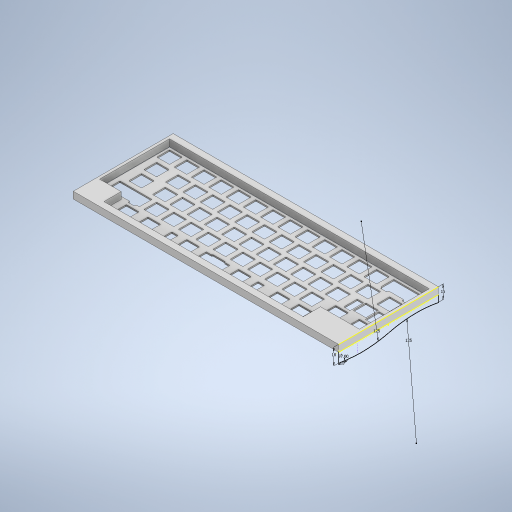
# Autodesk Inventor part: case
Saved by Autodesk Inventor 2023 (Build 270158000, 158)
## iProperties
Created: 2023-09-12
Part Number: case
Material: Generic
Document SubType Name: Modeling
Designer: Eric
Density: 1 g/cm^3
Appearance: Default
Author: Eric
Autodesk Inventor part; units mm, degrees
ref_plane "YZ Plane" through (0, 0, 0) normal (1, 0, 0) x (0, 1, 0)
ref_plane "XZ Plane" through (0, 0, 0) normal (0, 1, 0) x (-1, 0, 0)
ref_plane "XY Plane" through (0, 0, 0) normal (0, 0, 1) x (1, 0, 0)
sketch "Sketch1" plane through (0, 0, 0) normal (0, 1, 0) x (-1, 0, 0)
  line L0 (139.85, -45.1) -> (126.85, -45.1)
  line L1 (139.85, -31.1) -> (126.85, -31.1)
  line L2 (140.35, -44.6) -> (140.35, -31.6)
  line L3 (126.35, -44.6) -> (126.35, -31.6)
  arc A0 (139.85, -45.1) -> (140.35, -44.6) centre (139.85, -44.6) ccw
  arc A1 (126.35, -44.6) -> (126.85, -45.1) centre (126.85, -44.6) ccw
  arc A2 (140.35, -31.6) -> (139.85, -31.1) centre (139.85, -31.6) ccw
  arc A3 (126.85, -31.1) -> (126.35, -31.6) centre (126.85, -31.6) ccw
  line L4 (120.8, -45.1) -> (107.8, -45.1)
  line L5 (120.8, -31.1) -> (107.8, -31.1)
  line L6 (121.3, -44.6) -> (121.3, -31.6)
  line L7 (107.3, -44.6) -> (107.3, -31.6)
  arc A4 (120.8, -45.1) -> (121.3, -44.6) centre (120.8, -44.6) ccw
  arc A5 (107.3, -44.6) -> (107.8, -45.1) centre (107.8, -44.6) ccw
  arc A6 (121.3, -31.6) -> (120.8, -31.1) centre (120.8, -31.6) ccw
  arc A7 (107.8, -31.1) -> (107.3, -31.6) centre (107.8, -31.6) ccw
  line L8 (101.75, -45.1) -> (88.75, -45.1)
  line L9 (101.75, -31.1) -> (88.75, -31.1)
  line L10 (102.25, -44.6) -> (102.25, -31.6)
  line L11 (88.25, -44.6) -> (88.25, -31.6)
  arc A8 (101.75, -45.1) -> (102.25, -44.6) centre (101.75, -44.6) ccw
  arc A9 (88.25, -44.6) -> (88.75, -45.1) centre (88.75, -44.6) ccw
  arc A10 (102.25, -31.6) -> (101.75, -31.1) centre (101.75, -31.6) ccw
  arc A11 (88.75, -31.1) -> (88.25, -31.6) centre (88.75, -31.6) ccw
  line L12 (82.7, -45.1) -> (69.7, -45.1)
  line L13 (82.7, -31.1) -> (69.7, -31.1)
  line L14 (83.2, -44.6) -> (83.2, -31.6)
  line L15 (69.2, -44.6) -> (69.2, -31.6)
  arc A12 (82.7, -45.1) -> (83.2, -44.6) centre (82.7, -44.6) ccw
  arc A13 (69.2, -44.6) -> (69.7, -45.1) centre (69.7, -44.6) ccw
  arc A14 (83.2, -31.6) -> (82.7, -31.1) centre (82.7, -31.6) ccw
  arc A15 (69.7, -31.1) -> (69.2, -31.6) centre (69.7, -31.6) ccw
  line L16 (63.65, -45.1) -> (50.65, -45.1)
  line L17 (63.65, -31.1) -> (50.65, -31.1)
  line L18 (64.15, -44.6) -> (64.15, -31.6)
  line L19 (50.15, -44.6) -> (50.15, -31.6)
  arc A16 (63.65, -45.1) -> (64.15, -44.6) centre (63.65, -44.6) ccw
  arc A17 (50.15, -44.6) -> (50.65, -45.1) centre (50.65, -44.6) ccw
  arc A18 (64.15, -31.6) -> (63.65, -31.1) centre (63.65, -31.6) ccw
  arc A19 (50.65, -31.1) -> (50.15, -31.6) centre (50.65, -31.6) ccw
  line L20 (44.6, -45.1) -> (31.6, -45.1)
  line L21 (44.6, -31.1) -> (31.6, -31.1)
  line L22 (45.1, -44.6) -> (45.1, -31.6)
  line L23 (31.1, -44.6) -> (31.1, -31.6)
  arc A20 (44.6, -45.1) -> (45.1, -44.6) centre (44.6, -44.6) ccw
  arc A21 (31.1, -44.6) -> (31.6, -45.1) centre (31.6, -44.6) ccw
  arc A22 (45.1, -31.6) -> (44.6, -31.1) centre (44.6, -31.6) ccw
  arc A23 (31.6, -31.1) -> (31.1, -31.6) centre (31.6, -31.6) ccw
  line L24 (25.55, -45.1) -> (12.55, -45.1)
  line L25 (25.55, -31.1) -> (12.55, -31.1)
  line L26 (26.05, -44.6) -> (26.05, -31.6)
  line L27 (12.05, -44.6) -> (12.05, -31.6)
  arc A24 (25.55, -45.1) -> (26.05, -44.6) centre (25.55, -44.6) ccw
  arc A25 (12.05, -44.6) -> (12.55, -45.1) centre (12.55, -44.6) ccw
  arc A26 (26.05, -31.6) -> (25.55, -31.1) centre (25.55, -31.6) ccw
  arc A27 (12.55, -31.1) -> (12.05, -31.6) centre (12.55, -31.6) ccw
  line L28 (6.5, -45.1) -> (-6.5, -45.1)
  line L29 (6.5, -31.1) -> (-6.5, -31.1)
  line L30 (7, -44.6) -> (7, -31.6)
  line L31 (-7, -44.6) -> (-7, -31.6)
  arc A28 (6.5, -45.1) -> (7, -44.6) centre (6.5, -44.6) ccw
  arc A29 (-7, -44.6) -> (-6.5, -45.1) centre (-6.5, -44.6) ccw
  arc A30 (7, -31.6) -> (6.5, -31.1) centre (6.5, -31.6) ccw
  arc A31 (-6.5, -31.1) -> (-7, -31.6) centre (-6.5, -31.6) ccw
  line L32 (-12.55, -45.1) -> (-25.55, -45.1)
  line L33 (-12.55, -31.1) -> (-25.55, -31.1)
  line L34 (-12.05, -44.6) -> (-12.05, -31.6)
  line L35 (-26.05, -44.6) -> (-26.05, -31.6)
  arc A32 (-12.55, -45.1) -> (-12.05, -44.6) centre (-12.55, -44.6) ccw
  arc A33 (-26.05, -44.6) -> (-25.55, -45.1) centre (-25.55, -44.6) ccw
  arc A34 (-12.05, -31.6) -> (-12.55, -31.1) centre (-12.55, -31.6) ccw
  arc A35 (-25.55, -31.1) -> (-26.05, -31.6) centre (-25.55, -31.6) ccw
  line L36 (-31.6, -45.1) -> (-44.6, -45.1)
  line L37 (-31.6, -31.1) -> (-44.6, -31.1)
  line L38 (-31.1, -44.6) -> (-31.1, -31.6)
  line L39 (-45.1, -44.6) -> (-45.1, -31.6)
  arc A36 (-31.6, -45.1) -> (-31.1, -44.6) centre (-31.6, -44.6) ccw
  arc A37 (-45.1, -44.6) -> (-44.6, -45.1) centre (-44.6, -44.6) ccw
  arc A38 (-31.1, -31.6) -> (-31.6, -31.1) centre (-31.6, -31.6) ccw
  arc A39 (-44.6, -31.1) -> (-45.1, -31.6) centre (-44.6, -31.6) ccw
  line L40 (-50.65, -45.1) -> (-63.65, -45.1)
  line L41 (-50.65, -31.1) -> (-63.65, -31.1)
  line L42 (-50.15, -44.6) -> (-50.15, -31.6)
  line L43 (-64.15, -44.6) -> (-64.15, -31.6)
  arc A40 (-50.65, -45.1) -> (-50.15, -44.6) centre (-50.65, -44.6) ccw
  arc A41 (-64.15, -44.6) -> (-63.65, -45.1) centre (-63.65, -44.6) ccw
  arc A42 (-50.15, -31.6) -> (-50.65, -31.1) centre (-50.65, -31.6) ccw
  arc A43 (-63.65, -31.1) -> (-64.15, -31.6) centre (-63.65, -31.6) ccw
  line L44 (-69.7, -45.1) -> (-82.7, -45.1)
  line L45 (-69.7, -31.1) -> (-82.7, -31.1)
  line L46 (-69.2, -44.6) -> (-69.2, -31.6)
  line L47 (-83.2, -44.6) -> (-83.2, -31.6)
  arc A44 (-69.7, -45.1) -> (-69.2, -44.6) centre (-69.7, -44.6) ccw
  arc A45 (-83.2, -44.6) -> (-82.7, -45.1) centre (-82.7, -44.6) ccw
  arc A46 (-69.2, -31.6) -> (-69.7, -31.1) centre (-69.7, -31.6) ccw
  arc A47 (-82.7, -31.1) -> (-83.2, -31.6) centre (-82.7, -31.6) ccw
  line L48 (-88.75, -45.1) -> (-101.75, -45.1)
  line L49 (-88.75, -31.1) -> (-101.75, -31.1)
  line L50 (-88.25, -44.6) -> (-88.25, -31.6)
  line L51 (-102.25, -44.6) -> (-102.25, -31.6)
  arc A48 (-88.75, -45.1) -> (-88.25, -44.6) centre (-88.75, -44.6) ccw
  arc A49 (-102.25, -44.6) -> (-101.75, -45.1) centre (-101.75, -44.6) ccw
  arc A50 (-88.25, -31.6) -> (-88.75, -31.1) centre (-88.75, -31.6) ccw
  arc A51 (-101.75, -31.1) -> (-102.25, -31.6) centre (-101.75, -31.6) ccw
  line L52 (-117.325, -45.1) -> (-130.325, -45.1)
  line L53 (-117.325, -31.1) -> (-130.325, -31.1)
  line L54 (-108.887, -29.1) -> (-114.887, -29.1)
  line L55 (-108.387, -30.6) -> (-108.387, -29.6)
  line L56 (-115.387, -30.6) -> (-115.387, -29.6)
  arc A52 (-108.387, -29.6) -> (-108.887, -29.1) centre (-108.887, -29.6) ccw
  arc A53 (-114.887, -29.1) -> (-115.387, -29.6) centre (-114.887, -29.6) ccw
  line L57 (-132.763, -29.1) -> (-138.763, -29.1)
  line L58 (-132.263, -30.6) -> (-132.263, -29.6)
  line L59 (-139.263, -30.6) -> (-139.263, -29.6)
  arc A54 (-132.263, -29.6) -> (-132.763, -29.1) centre (-132.763, -29.6) ccw
  arc A55 (-138.763, -29.1) -> (-139.263, -29.6) centre (-138.763, -29.6) ccw
  line L60 (-107.8, -45.1) -> (-120.8, -45.1)
  line L61 (-107.3, -44.6) -> (-107.3, -31.6)
  arc A56 (-107.8, -45.1) -> (-107.3, -44.6) centre (-107.8, -44.6) ccw
  arc A57 (-107.3, -31.6) -> (-107.8, -31.1) centre (-107.8, -31.6) ccw
  line L62 (-126.85, -45.1) -> (-139.85, -45.1)
  line L63 (-140.35, -44.6) -> (-140.35, -31.6)
  arc A58 (-140.35, -44.6) -> (-139.85, -45.1) centre (-139.85, -44.6) ccw
  arc A59 (-139.85, -31.1) -> (-140.35, -31.6) centre (-139.85, -31.6) ccw
  line L64 (135.0875, -26.05) -> (122.0875, -26.05)
  line L65 (135.0875, -12.05) -> (122.0875, -12.05)
  line L66 (135.5875, -25.55) -> (135.5875, -12.55)
  line L67 (121.5875, -25.55) -> (121.5875, -12.55)
  arc A60 (135.0875, -26.05) -> (135.5875, -25.55) centre (135.0875, -25.55) ccw
  arc A61 (121.5875, -25.55) -> (122.0875, -26.05) centre (122.0875, -25.55) ccw
  arc A62 (135.5875, -12.55) -> (135.0875, -12.05) centre (135.0875, -12.55) ccw
  arc A63 (122.0875, -12.05) -> (121.5875, -12.55) centre (122.0875, -12.55) ccw
  line L68 (111.275, -26.05) -> (98.275, -26.05)
  line L69 (111.275, -12.05) -> (98.275, -12.05)
  line L70 (111.775, -25.55) -> (111.775, -12.55)
  line L71 (97.775, -25.55) -> (97.775, -12.55)
  arc A64 (111.275, -26.05) -> (111.775, -25.55) centre (111.275, -25.55) ccw
  arc A65 (97.775, -25.55) -> (98.275, -26.05) centre (98.275, -25.55) ccw
  arc A66 (111.775, -12.55) -> (111.275, -12.05) centre (111.275, -12.55) ccw
  arc A67 (98.275, -12.05) -> (97.775, -12.55) centre (98.275, -12.55) ccw
  line L72 (92.225, -26.05) -> (79.225, -26.05)
  line L73 (92.225, -12.05) -> (79.225, -12.05)
  line L74 (92.725, -25.55) -> (92.725, -12.55)
  line L75 (78.725, -25.55) -> (78.725, -12.55)
  arc A68 (92.225, -26.05) -> (92.725, -25.55) centre (92.225, -25.55) ccw
  arc A69 (78.725, -25.55) -> (79.225, -26.05) centre (79.225, -25.55) ccw
  arc A70 (92.725, -12.55) -> (92.225, -12.05) centre (92.225, -12.55) ccw
  arc A71 (79.225, -12.05) -> (78.725, -12.55) centre (79.225, -12.55) ccw
  line L76 (73.175, -26.05) -> (60.175, -26.05)
  line L77 (73.175, -12.05) -> (60.175, -12.05)
  line L78 (73.675, -25.55) -> (73.675, -12.55)
  line L79 (59.675, -25.55) -> (59.675, -12.55)
  arc A72 (73.175, -26.05) -> (73.675, -25.55) centre (73.175, -25.55) ccw
  arc A73 (59.675, -25.55) -> (60.175, -26.05) centre (60.175, -25.55) ccw
  arc A74 (73.675, -12.55) -> (73.175, -12.05) centre (73.175, -12.55) ccw
  arc A75 (60.175, -12.05) -> (59.675, -12.55) centre (60.175, -12.55) ccw
  line L80 (54.125, -26.05) -> (41.125, -26.05)
  line L81 (54.125, -12.05) -> (41.125, -12.05)
  line L82 (54.625, -25.55) -> (54.625, -12.55)
  line L83 (40.625, -25.55) -> (40.625, -12.55)
  arc A76 (54.125, -26.05) -> (54.625, -25.55) centre (54.125, -25.55) ccw
  arc A77 (40.625, -25.55) -> (41.125, -26.05) centre (41.125, -25.55) ccw
  arc A78 (54.625, -12.55) -> (54.125, -12.05) centre (54.125, -12.55) ccw
  arc A79 (41.125, -12.05) -> (40.625, -12.55) centre (41.125, -12.55) ccw
  line L84 (35.075, -26.05) -> (22.075, -26.05)
  line L85 (35.075, -12.05) -> (22.075, -12.05)
  line L86 (35.575, -25.55) -> (35.575, -12.55)
  line L87 (21.575, -25.55) -> (21.575, -12.55)
  arc A80 (35.075, -26.05) -> (35.575, -25.55) centre (35.075, -25.55) ccw
  arc A81 (21.575, -25.55) -> (22.075, -26.05) centre (22.075, -25.55) ccw
  arc A82 (35.575, -12.55) -> (35.075, -12.05) centre (35.075, -12.55) ccw
  arc A83 (22.075, -12.05) -> (21.575, -12.55) centre (22.075, -12.55) ccw
  line L88 (16.025, -26.05) -> (3.025, -26.05)
  line L89 (16.025, -12.05) -> (3.025, -12.05)
  line L90 (16.525, -25.55) -> (16.525, -12.55)
  line L91 (2.525, -25.55) -> (2.525, -12.55)
  arc A84 (16.025, -26.05) -> (16.525, -25.55) centre (16.025, -25.55) ccw
  arc A85 (2.525, -25.55) -> (3.025, -26.05) centre (3.025, -25.55) ccw
  arc A86 (16.525, -12.55) -> (16.025, -12.05) centre (16.025, -12.55) ccw
  arc A87 (3.025, -12.05) -> (2.525, -12.55) centre (3.025, -12.55) ccw
  line L92 (-3.025, -26.05) -> (-16.025, -26.05)
  line L93 (-3.025, -12.05) -> (-16.025, -12.05)
  line L94 (-2.525, -25.55) -> (-2.525, -12.55)
  line L95 (-16.525, -25.55) -> (-16.525, -12.55)
  arc A88 (-3.025, -26.05) -> (-2.525, -25.55) centre (-3.025, -25.55) ccw
  arc A89 (-16.525, -25.55) -> (-16.025, -26.05) centre (-16.025, -25.55) ccw
  arc A90 (-2.525, -12.55) -> (-3.025, -12.05) centre (-3.025, -12.55) ccw
  arc A91 (-16.025, -12.05) -> (-16.525, -12.55) centre (-16.025, -12.55) ccw
  line L96 (-22.075, -26.05) -> (-35.075, -26.05)
  line L97 (-22.075, -12.05) -> (-35.075, -12.05)
  line L98 (-21.575, -25.55) -> (-21.575, -12.55)
  line L99 (-35.575, -25.55) -> (-35.575, -12.55)
  arc A92 (-22.075, -26.05) -> (-21.575, -25.55) centre (-22.075, -25.55) ccw
  arc A93 (-35.575, -25.55) -> (-35.075, -26.05) centre (-35.075, -25.55) ccw
  arc A94 (-21.575, -12.55) -> (-22.075, -12.05) centre (-22.075, -12.55) ccw
  arc A95 (-35.075, -12.05) -> (-35.575, -12.55) centre (-35.075, -12.55) ccw
  line L100 (-41.125, -26.05) -> (-54.125, -26.05)
  line L101 (-41.125, -12.05) -> (-54.125, -12.05)
  line L102 (-40.625, -25.55) -> (-40.625, -12.55)
  line L103 (-54.625, -25.55) -> (-54.625, -12.55)
  arc A96 (-41.125, -26.05) -> (-40.625, -25.55) centre (-41.125, -25.55) ccw
  arc A97 (-54.625, -25.55) -> (-54.125, -26.05) centre (-54.125, -25.55) ccw
  arc A98 (-40.625, -12.55) -> (-41.125, -12.05) centre (-41.125, -12.55) ccw
  arc A99 (-54.125, -12.05) -> (-54.625, -12.55) centre (-54.125, -12.55) ccw
  line L104 (-60.175, -26.05) -> (-73.175, -26.05)
  line L105 (-60.175, -12.05) -> (-73.175, -12.05)
  line L106 (-59.675, -25.55) -> (-59.675, -12.55)
  line L107 (-73.675, -25.55) -> (-73.675, -12.55)
  arc A100 (-60.175, -26.05) -> (-59.675, -25.55) centre (-60.175, -25.55) ccw
  arc A101 (-73.675, -25.55) -> (-73.175, -26.05) centre (-73.175, -25.55) ccw
  arc A102 (-59.675, -12.55) -> (-60.175, -12.05) centre (-60.175, -12.55) ccw
  arc A103 (-73.175, -12.05) -> (-73.675, -12.55) centre (-73.175, -12.55) ccw
  line L108 (-79.225, -26.05) -> (-92.225, -26.05)
  line L109 (-79.225, -12.05) -> (-92.225, -12.05)
  line L110 (-78.725, -25.55) -> (-78.725, -12.55)
  line L111 (-92.725, -25.55) -> (-92.725, -12.55)
  arc A104 (-79.225, -26.05) -> (-78.725, -25.55) centre (-79.225, -25.55) ccw
  arc A105 (-92.725, -25.55) -> (-92.225, -26.05) centre (-92.225, -25.55) ccw
  arc A106 (-78.725, -12.55) -> (-79.225, -12.05) centre (-79.225, -12.55) ccw
  arc A107 (-92.225, -12.05) -> (-92.725, -12.55) centre (-92.225, -12.55) ccw
  line L112 (-98.275, -26.05) -> (-111.275, -26.05)
  line L113 (-98.275, -12.05) -> (-111.275, -12.05)
  line L114 (-97.775, -25.55) -> (-97.775, -12.55)
  line L115 (-111.775, -25.55) -> (-111.775, -12.55)
  arc A108 (-98.275, -26.05) -> (-97.775, -25.55) centre (-98.275, -25.55) ccw
  arc A109 (-111.775, -25.55) -> (-111.275, -26.05) centre (-111.275, -25.55) ccw
  arc A110 (-97.775, -12.55) -> (-98.275, -12.05) centre (-98.275, -12.55) ccw
  arc A111 (-111.275, -12.05) -> (-111.775, -12.55) centre (-111.275, -12.55) ccw
  line L116 (-122.0875, -26.05) -> (-135.0875, -26.05)
  line L117 (-122.0875, -12.05) -> (-135.0875, -12.05)
  line L118 (-121.5875, -25.55) -> (-121.5875, -12.55)
  line L119 (-135.5875, -25.55) -> (-135.5875, -12.55)
  arc A112 (-122.0875, -26.05) -> (-121.5875, -25.55) centre (-122.0875, -25.55) ccw
  arc A113 (-135.5875, -25.55) -> (-135.0875, -26.05) centre (-135.0875, -25.55) ccw
  arc A114 (-121.5875, -12.55) -> (-122.0875, -12.05) centre (-122.0875, -12.55) ccw
  arc A115 (-135.0875, -12.05) -> (-135.5875, -12.55) centre (-135.0875, -12.55) ccw
  line L120 (132.7062, -7) -> (119.7062, -7)
  line L121 (132.7062, 7) -> (119.7062, 7)
  line L122 (133.2062, -6.5) -> (133.2062, 6.5)
  line L123 (119.2062, -6.5) -> (119.2062, 6.5)
  arc A116 (132.7062, -7) -> (133.2062, -6.5) centre (132.7062, -6.5) ccw
  arc A117 (119.2062, -6.5) -> (119.7062, -7) centre (119.7062, -6.5) ccw
  arc A118 (133.2062, 6.5) -> (132.7062, 7) centre (132.7062, 6.5) ccw
  arc A119 (119.7062, 7) -> (119.2062, 6.5) centre (119.7062, 6.5) ccw
  line L124 (106.5125, -7) -> (93.5125, -7)
  line L125 (106.5125, 7) -> (93.5125, 7)
  line L126 (107.0125, -6.5) -> (107.0125, 6.5)
  line L127 (93.0125, -6.5) -> (93.0125, 6.5)
  arc A120 (106.5125, -7) -> (107.0125, -6.5) centre (106.5125, -6.5) ccw
  arc A121 (93.0125, -6.5) -> (93.5125, -7) centre (93.5125, -6.5) ccw
  arc A122 (107.0125, 6.5) -> (106.5125, 7) centre (106.5125, 6.5) ccw
  arc A123 (93.5125, 7) -> (93.0125, 6.5) centre (93.5125, 6.5) ccw
  line L128 (87.4625, -7) -> (74.4625, -7)
  line L129 (87.4625, 7) -> (74.4625, 7)
  line L130 (87.9625, -6.5) -> (87.9625, 6.5)
  line L131 (73.9625, -6.5) -> (73.9625, 6.5)
  arc A124 (87.4625, -7) -> (87.9625, -6.5) centre (87.4625, -6.5) ccw
  arc A125 (73.9625, -6.5) -> (74.4625, -7) centre (74.4625, -6.5) ccw
  arc A126 (87.9625, 6.5) -> (87.4625, 7) centre (87.4625, 6.5) ccw
  arc A127 (74.4625, 7) -> (73.9625, 6.5) centre (74.4625, 6.5) ccw
  line L132 (68.4125, -7) -> (55.4125, -7)
  line L133 (68.4125, 7) -> (55.4125, 7)
  line L134 (68.9125, -6.5) -> (68.9125, 6.5)
  line L135 (54.9125, -6.5) -> (54.9125, 6.5)
  arc A128 (68.4125, -7) -> (68.9125, -6.5) centre (68.4125, -6.5) ccw
  arc A129 (54.9125, -6.5) -> (55.4125, -7) centre (55.4125, -6.5) ccw
  arc A130 (68.9125, 6.5) -> (68.4125, 7) centre (68.4125, 6.5) ccw
  arc A131 (55.4125, 7) -> (54.9125, 6.5) centre (55.4125, 6.5) ccw
  line L136 (49.3625, -7) -> (36.3625, -7)
  line L137 (49.3625, 7) -> (36.3625, 7)
  line L138 (49.8625, -6.5) -> (49.8625, 6.5)
  line L139 (35.8625, -6.5) -> (35.8625, 6.5)
  arc A132 (49.3625, -7) -> (49.8625, -6.5) centre (49.3625, -6.5) ccw
  arc A133 (35.8625, -6.5) -> (36.3625, -7) centre (36.3625, -6.5) ccw
  arc A134 (49.8625, 6.5) -> (49.3625, 7) centre (49.3625, 6.5) ccw
  arc A135 (36.3625, 7) -> (35.8625, 6.5) centre (36.3625, 6.5) ccw
  line L140 (30.3125, -7) -> (17.3125, -7)
  line L141 (30.3125, 7) -> (17.3125, 7)
  line L142 (30.8125, -6.5) -> (30.8125, 6.5)
  line L143 (16.8125, -6.5) -> (16.8125, 6.5)
  arc A136 (30.3125, -7) -> (30.8125, -6.5) centre (30.3125, -6.5) ccw
  arc A137 (16.8125, -6.5) -> (17.3125, -7) centre (17.3125, -6.5) ccw
  arc A138 (30.8125, 6.5) -> (30.3125, 7) centre (30.3125, 6.5) ccw
  arc A139 (17.3125, 7) -> (16.8125, 6.5) centre (17.3125, 6.5) ccw
  line L144 (11.2625, -7) -> (-1.7375, -7)
  line L145 (11.2625, 7) -> (-1.7375, 7)
  line L146 (11.7625, -6.5) -> (11.7625, 6.5)
  line L147 (-2.2375, -6.5) -> (-2.2375, 6.5)
  arc A140 (11.2625, -7) -> (11.7625, -6.5) centre (11.2625, -6.5) ccw
  arc A141 (-2.2375, -6.5) -> (-1.7375, -7) centre (-1.7375, -6.5) ccw
  arc A142 (11.7625, 6.5) -> (11.2625, 7) centre (11.2625, 6.5) ccw
  arc A143 (-1.7375, 7) -> (-2.2375, 6.5) centre (-1.7375, 6.5) ccw
  line L148 (-7.7875, -7) -> (-20.7875, -7)
  line L149 (-7.7875, 7) -> (-20.7875, 7)
  line L150 (-7.2875, -6.5) -> (-7.2875, 6.5)
  line L151 (-21.2875, -6.5) -> (-21.2875, 6.5)
  arc A144 (-7.7875, -7) -> (-7.2875, -6.5) centre (-7.7875, -6.5) ccw
  arc A145 (-21.2875, -6.5) -> (-20.7875, -7) centre (-20.7875, -6.5) ccw
  arc A146 (-7.2875, 6.5) -> (-7.7875, 7) centre (-7.7875, 6.5) ccw
  arc A147 (-20.7875, 7) -> (-21.2875, 6.5) centre (-20.7875, 6.5) ccw
  line L152 (-26.8375, -7) -> (-39.8375, -7)
  line L153 (-26.8375, 7) -> (-39.8375, 7)
  line L154 (-26.3375, -6.5) -> (-26.3375, 6.5)
  line L155 (-40.3375, -6.5) -> (-40.3375, 6.5)
  arc A148 (-26.8375, -7) -> (-26.3375, -6.5) centre (-26.8375, -6.5) ccw
  arc A149 (-40.3375, -6.5) -> (-39.8375, -7) centre (-39.8375, -6.5) ccw
  arc A150 (-26.3375, 6.5) -> (-26.8375, 7) centre (-26.8375, 6.5) ccw
  arc A151 (-39.8375, 7) -> (-40.3375, 6.5) centre (-39.8375, 6.5) ccw
  line L156 (-45.8875, -7) -> (-58.8875, -7)
  line L157 (-45.8875, 7) -> (-58.8875, 7)
  line L158 (-45.3875, -6.5) -> (-45.3875, 6.5)
  line L159 (-59.3875, -6.5) -> (-59.3875, 6.5)
  arc A152 (-45.8875, -7) -> (-45.3875, -6.5) centre (-45.8875, -6.5) ccw
  arc A153 (-59.3875, -6.5) -> (-58.8875, -7) centre (-58.8875, -6.5) ccw
  arc A154 (-45.3875, 6.5) -> (-45.8875, 7) centre (-45.8875, 6.5) ccw
  arc A155 (-58.8875, 7) -> (-59.3875, 6.5) centre (-58.8875, 6.5) ccw
  line L160 (-64.9375, -7) -> (-77.9375, -7)
  line L161 (-64.9375, 7) -> (-77.9375, 7)
  line L162 (-64.4375, -6.5) -> (-64.4375, 6.5)
  line L163 (-78.4375, -6.5) -> (-78.4375, 6.5)
  arc A156 (-64.9375, -7) -> (-64.4375, -6.5) centre (-64.9375, -6.5) ccw
  arc A157 (-78.4375, -6.5) -> (-77.9375, -7) centre (-77.9375, -6.5) ccw
  arc A158 (-64.4375, 6.5) -> (-64.9375, 7) centre (-64.9375, 6.5) ccw
  arc A159 (-77.9375, 7) -> (-78.4375, 6.5) centre (-77.9375, 6.5) ccw
  line L164 (-83.9875, -7) -> (-96.9875, -7)
  line L165 (-83.9875, 7) -> (-96.9875, 7)
  line L166 (-83.4875, -6.5) -> (-83.4875, 6.5)
  line L167 (-97.4875, -6.5) -> (-97.4875, 6.5)
  arc A160 (-83.9875, -7) -> (-83.4875, -6.5) centre (-83.9875, -6.5) ccw
  arc A161 (-97.4875, -6.5) -> (-96.9875, -7) centre (-96.9875, -6.5) ccw
  arc A162 (-83.4875, 6.5) -> (-83.9875, 7) centre (-83.9875, 6.5) ccw
  arc A163 (-96.9875, 7) -> (-97.4875, 6.5) centre (-96.9875, 6.5) ccw
  line L168 (-114.9438, -7) -> (-127.9438, -7)
  line L169 (-114.9437, 7) -> (-127.9437, 7)
  line L170 (-114.4438, -6.5) -> (-114.4437, 6.5)
  line L171 (-128.4438, -6.5) -> (-128.4438, 6.5)
  arc A164 (-114.9438, -7) -> (-114.4438, -6.5) centre (-114.9438, -6.5) ccw
  arc A165 (-128.4438, -6.5) -> (-127.9438, -7) centre (-127.9438, -6.5) ccw
  arc A166 (-114.4437, 6.5) -> (-114.9437, 7) centre (-114.9437, 6.5) ccw
  arc A167 (-127.9437, 7) -> (-128.4438, 6.5) centre (-127.9438, 6.5) ccw
  line L172 (-106.5058, -6) -> (-112.5058, -6)
  line L173 (-106.5058, 9) -> (-112.5057, 9)
  line L174 (-106.0058, -5.5) -> (-106.0058, 8.5)
  line L175 (-113.0058, -5.5) -> (-113.0057, 8.5)
  arc A168 (-106.5058, -6) -> (-106.0058, -5.5) centre (-106.5058, -5.5) ccw
  arc A169 (-113.0058, -5.5) -> (-112.5058, -6) centre (-112.5058, -5.5) ccw
  arc A170 (-106.0058, 8.5) -> (-106.5058, 9) centre (-106.5058, 8.5) ccw
  arc A171 (-112.5057, 9) -> (-113.0057, 8.5) centre (-112.5057, 8.5) ccw
  line L176 (-130.3817, -6) -> (-136.3817, -6)
  line L177 (-130.3818, 9) -> (-136.3818, 9)
  line L178 (-129.8818, -5.5) -> (-129.8818, 8.5)
  line L179 (-136.8817, -5.5) -> (-136.8818, 8.5)
  arc A172 (-130.3817, -6) -> (-129.8818, -5.5) centre (-130.3818, -5.5) ccw
  arc A173 (-136.8817, -5.5) -> (-136.3817, -6) centre (-136.3817, -5.5) ccw
  arc A174 (-129.8818, 8.5) -> (-130.3818, 9) centre (-130.3818, 8.5) ccw
  arc A175 (-136.3818, 9) -> (-136.8818, 8.5) centre (-136.3818, 8.5) ccw
  line L180 (127.9437, 12.05) -> (114.9437, 12.05)
  line L181 (127.9437, 26.05) -> (114.9437, 26.05)
  line L182 (136.3817, 28.05) -> (130.3817, 28.05)
  line L183 (136.8817, 26.55) -> (136.8817, 27.55)
  line L184 (129.8817, 26.55) -> (129.8817, 27.55)
  arc A176 (136.8817, 27.55) -> (136.3817, 28.05) centre (136.3817, 27.55) ccw
  arc A177 (130.3817, 28.05) -> (129.8817, 27.55) centre (130.3817, 27.55) ccw
  line L185 (112.5057, 28.05) -> (106.5058, 28.05)
  line L186 (113.0057, 26.55) -> (113.0057, 27.55)
  line L187 (106.0057, 26.55) -> (106.0057, 27.55)
  arc A178 (113.0057, 27.55) -> (112.5057, 28.05) centre (112.5057, 27.55) ccw
  arc A179 (106.5058, 28.05) -> (106.0057, 27.55) centre (106.5058, 27.55) ccw
  line L188 (137.4688, 12.05) -> (124.4687, 12.05)
  line L189 (137.9687, 12.55) -> (137.9687, 25.55)
  arc A180 (137.4688, 12.05) -> (137.9687, 12.55) centre (137.4687, 12.55) ccw
  arc A181 (137.9687, 25.55) -> (137.4688, 26.05) centre (137.4688, 25.55) ccw
  line L190 (116.0375, 12.05) -> (103.0375, 12.05)
  line L191 (102.5375, 12.55) -> (102.5375, 25.55)
  arc A182 (102.5375, 12.55) -> (103.0375, 12.05) centre (103.0375, 12.55) ccw
  arc A183 (103.0375, 26.05) -> (102.5375, 25.55) centre (103.0375, 25.55) ccw
  line L192 (96.9875, 12.05) -> (83.9875, 12.05)
  line L193 (96.9875, 26.05) -> (83.9875, 26.05)
  line L194 (97.4875, 12.55) -> (97.4875, 25.55)
  line L195 (83.4875, 12.55) -> (83.4875, 25.55)
  arc A184 (96.9875, 12.05) -> (97.4875, 12.55) centre (96.9875, 12.55) ccw
  arc A185 (83.4875, 12.55) -> (83.9875, 12.05) centre (83.9875, 12.55) ccw
  arc A186 (97.4875, 25.55) -> (96.9875, 26.05) centre (96.9875, 25.55) ccw
  arc A187 (83.9875, 26.05) -> (83.4875, 25.55) centre (83.9875, 25.55) ccw
  line L196 (77.9375, 12.05) -> (64.9375, 12.05)
  line L197 (77.9375, 26.05) -> (64.9375, 26.05)
  line L198 (78.4375, 12.55) -> (78.4375, 25.55)
  line L199 (64.4375, 12.55) -> (64.4375, 25.55)
  arc A188 (77.9375, 12.05) -> (78.4375, 12.55) centre (77.9375, 12.55) ccw
  arc A189 (64.4375, 12.55) -> (64.9375, 12.05) centre (64.9375, 12.55) ccw
  arc A190 (78.4375, 25.55) -> (77.9375, 26.05) centre (77.9375, 25.55) ccw
  arc A191 (64.9375, 26.05) -> (64.4375, 25.55) centre (64.9375, 25.55) ccw
  line L200 (58.8875, 12.05) -> (45.8875, 12.05)
  line L201 (58.8875, 26.05) -> (45.8875, 26.05)
  line L202 (59.3875, 12.55) -> (59.3875, 25.55)
  line L203 (45.3875, 12.55) -> (45.3875, 25.55)
  arc A192 (58.8875, 12.05) -> (59.3875, 12.55) centre (58.8875, 12.55) ccw
  arc A193 (45.3875, 12.55) -> (45.8875, 12.05) centre (45.8875, 12.55) ccw
  arc A194 (59.3875, 25.55) -> (58.8875, 26.05) centre (58.8875, 25.55) ccw
  arc A195 (45.8875, 26.05) -> (45.3875, 25.55) centre (45.8875, 25.55) ccw
  line L204 (39.8375, 12.05) -> (26.8375, 12.05)
  line L205 (39.8375, 26.05) -> (26.8375, 26.05)
  line L206 (40.3375, 12.55) -> (40.3375, 25.55)
  line L207 (26.3375, 12.55) -> (26.3375, 25.55)
  arc A196 (39.8375, 12.05) -> (40.3375, 12.55) centre (39.8375, 12.55) ccw
  arc A197 (26.3375, 12.55) -> (26.8375, 12.05) centre (26.8375, 12.55) ccw
  arc A198 (40.3375, 25.55) -> (39.8375, 26.05) centre (39.8375, 25.55) ccw
  arc A199 (26.8375, 26.05) -> (26.3375, 25.55) centre (26.8375, 25.55) ccw
  line L208 (20.7875, 12.05) -> (7.7875, 12.05)
  line L209 (20.7875, 26.05) -> (7.7875, 26.05)
  line L210 (21.2875, 12.55) -> (21.2875, 25.55)
  line L211 (7.2875, 12.55) -> (7.2875, 25.55)
  arc A200 (20.7875, 12.05) -> (21.2875, 12.55) centre (20.7875, 12.55) ccw
  arc A201 (7.2875, 12.55) -> (7.7875, 12.05) centre (7.7875, 12.55) ccw
  arc A202 (21.2875, 25.55) -> (20.7875, 26.05) centre (20.7875, 25.55) ccw
  arc A203 (7.7875, 26.05) -> (7.2875, 25.55) centre (7.7875, 25.55) ccw
  line L212 (1.7375, 12.05) -> (-11.2625, 12.05)
  line L213 (1.7375, 26.05) -> (-11.2625, 26.05)
  line L214 (2.2375, 12.55) -> (2.2375, 25.55)
  line L215 (-11.7625, 12.55) -> (-11.7625, 25.55)
  arc A204 (1.7375, 12.05) -> (2.2375, 12.55) centre (1.7375, 12.55) ccw
  arc A205 (-11.7625, 12.55) -> (-11.2625, 12.05) centre (-11.2625, 12.55) ccw
  arc A206 (2.2375, 25.55) -> (1.7375, 26.05) centre (1.7375, 25.55) ccw
  arc A207 (-11.2625, 26.05) -> (-11.7625, 25.55) centre (-11.2625, 25.55) ccw
  line L216 (-17.3125, 12.05) -> (-30.3125, 12.05)
  line L217 (-17.3125, 26.05) -> (-30.3125, 26.05)
  line L218 (-16.8125, 12.55) -> (-16.8125, 25.55)
  line L219 (-30.8125, 12.55) -> (-30.8125, 25.55)
  arc A208 (-17.3125, 12.05) -> (-16.8125, 12.55) centre (-17.3125, 12.55) ccw
  arc A209 (-30.8125, 12.55) -> (-30.3125, 12.05) centre (-30.3125, 12.55) ccw
  arc A210 (-16.8125, 25.55) -> (-17.3125, 26.05) centre (-17.3125, 25.55) ccw
  arc A211 (-30.3125, 26.05) -> (-30.8125, 25.55) centre (-30.3125, 25.55) ccw
  line L220 (-36.3625, 12.05) -> (-49.3625, 12.05)
  line L221 (-36.3625, 26.05) -> (-49.3625, 26.05)
  line L222 (-35.8625, 12.55) -> (-35.8625, 25.55)
  line L223 (-49.8625, 12.55) -> (-49.8625, 25.55)
  arc A212 (-36.3625, 12.05) -> (-35.8625, 12.55) centre (-36.3625, 12.55) ccw
  arc A213 (-49.8625, 12.55) -> (-49.3625, 12.05) centre (-49.3625, 12.55) ccw
  arc A214 (-35.8625, 25.55) -> (-36.3625, 26.05) centre (-36.3625, 25.55) ccw
  arc A215 (-49.3625, 26.05) -> (-49.8625, 25.55) centre (-49.3625, 25.55) ccw
  line L224 (-55.4125, 12.05) -> (-68.4125, 12.05)
  line L225 (-55.4125, 26.05) -> (-68.4125, 26.05)
  line L226 (-54.9125, 12.55) -> (-54.9125, 25.55)
  line L227 (-68.9125, 12.55) -> (-68.9125, 25.55)
  arc A216 (-55.4125, 12.05) -> (-54.9125, 12.55) centre (-55.4125, 12.55) ccw
  arc A217 (-68.9125, 12.55) -> (-68.4125, 12.05) centre (-68.4125, 12.55) ccw
  arc A218 (-54.9125, 25.55) -> (-55.4125, 26.05) centre (-55.4125, 25.55) ccw
  arc A219 (-68.4125, 26.05) -> (-68.9125, 25.55) centre (-68.4125, 25.55) ccw
  line L228 (-74.4625, 12.05) -> (-87.4625, 12.05)
  line L229 (-74.4625, 26.05) -> (-87.4625, 26.05)
  line L230 (-73.9625, 12.55) -> (-73.9625, 25.55)
  line L231 (-87.9625, 12.55) -> (-87.9625, 25.55)
  arc A220 (-74.4625, 12.05) -> (-73.9625, 12.55) centre (-74.4625, 12.55) ccw
  arc A221 (-87.9625, 12.55) -> (-87.4625, 12.05) centre (-87.4625, 12.55) ccw
  arc A222 (-73.9625, 25.55) -> (-74.4625, 26.05) centre (-74.4625, 25.55) ccw
  arc A223 (-87.4625, 26.05) -> (-87.9625, 25.55) centre (-87.4625, 25.55) ccw
  line L232 (-100.6562, 12.05) -> (-113.6563, 12.05)
  line L233 (-100.6562, 26.05) -> (-113.6562, 26.05)
  line L234 (-100.1563, 12.55) -> (-100.1562, 25.55)
  line L235 (-114.1563, 12.55) -> (-114.1562, 25.55)
  arc A224 (-100.6562, 12.05) -> (-100.1563, 12.55) centre (-100.6563, 12.55) ccw
  arc A225 (-114.1563, 12.55) -> (-113.6563, 12.05) centre (-113.6563, 12.55) ccw
  arc A226 (-100.1562, 25.55) -> (-100.6562, 26.05) centre (-100.6562, 25.55) ccw
  arc A227 (-113.6562, 26.05) -> (-114.1562, 25.55) centre (-113.6562, 25.55) ccw
  line L236 (-126.85, 12.05) -> (-139.85, 12.05)
  line L237 (-126.85, 26.05) -> (-139.85, 26.05)
  line L238 (-126.35, 12.55) -> (-126.35, 25.55)
  line L239 (-140.35, 12.55) -> (-140.35, 25.55)
  arc A228 (-126.85, 12.05) -> (-126.35, 12.55) centre (-126.85, 12.55) ccw
  arc A229 (-140.35, 12.55) -> (-139.85, 12.05) centre (-139.85, 12.55) ccw
  arc A230 (-126.35, 25.55) -> (-126.85, 26.05) centre (-126.85, 25.55) ccw
  arc A231 (-139.85, 26.05) -> (-140.35, 25.55) centre (-139.85, 25.55) ccw
  line L240 (111.275, 31.1) -> (98.275, 31.1)
  line L241 (111.275, 45.1) -> (98.275, 45.1)
  line L242 (111.775, 31.6) -> (111.775, 44.6)
  line L243 (97.775, 31.6) -> (97.775, 44.6)
  arc A232 (111.275, 31.1) -> (111.775, 31.6) centre (111.275, 31.6) ccw
  arc A233 (97.775, 31.6) -> (98.275, 31.1) centre (98.275, 31.6) ccw
  arc A234 (111.775, 44.6) -> (111.275, 45.1) centre (111.275, 44.6) ccw
  arc A235 (98.275, 45.1) -> (97.775, 44.6) centre (98.275, 44.6) ccw
  line L244 (87.4625, 31.1) -> (74.4625, 31.1)
  line L245 (87.4625, 45.1) -> (74.4625, 45.1)
  line L246 (87.9625, 31.6) -> (87.9625, 44.6)
  line L247 (73.9625, 31.6) -> (73.9625, 44.6)
  arc A236 (87.4625, 31.1) -> (87.9625, 31.6) centre (87.4625, 31.6) ccw
  arc A237 (73.9625, 31.6) -> (74.4625, 31.1) centre (74.4625, 31.6) ccw
  arc A238 (87.9625, 44.6) -> (87.4625, 45.1) centre (87.4625, 44.6) ccw
  arc A239 (74.4625, 45.1) -> (73.9625, 44.6) centre (74.4625, 44.6) ccw
  line L248 (16.025, 31.1) -> (3.025, 31.1)
  line L249 (15.05, 45.1) -> (4, 45.1)
  line L250 (16.525, 31.6) -> (16.525, 31.6)
  line L251 (2.525, 31.6) -> (2.525, 31.6)
  arc A240 (16.025, 31.1) -> (16.525, 31.6) centre (16.025, 31.6) ccw
  arc A241 (2.525, 31.6) -> (3.025, 31.1) centre (3.025, 31.6) ccw
  line L252 (60.15, 32.1) -> (54.15, 32.1)
  line L253 (60.65, 32.6) -> (60.65, 45.625)
  line L254 (53.65, 32.6) -> (53.65, 45.625)
  arc A242 (60.15, 32.1) -> (60.65, 32.6) centre (60.15, 32.6) ccw
  arc A243 (53.65, 32.6) -> (54.15, 32.1) centre (54.15, 32.6) ccw
  line L255 (-35.1, 32.1) -> (-41.1, 32.1)
  line L256 (-34.6, 32.6) -> (-34.6, 45.625)
  line L257 (-41.6, 32.6) -> (-41.6, 45.625)
  arc A244 (-35.1, 32.1) -> (-34.6, 32.6) centre (-35.1, 32.6) ccw
  arc A245 (-41.6, 32.6) -> (-41.1, 32.1) centre (-41.1, 32.6) ccw
  line L258 (44.6, 31.1) -> (31.6, 31.1)
  line L259 (44.6, 45.1) -> (31.6, 45.1)
  line L260 (45.1, 31.6) -> (45.1, 44.6)
  line L261 (31.1, 31.6) -> (31.1, 44.6)
  arc A246 (44.6, 31.1) -> (45.1, 31.6) centre (44.6, 31.6) ccw
  arc A247 (31.1, 31.6) -> (31.6, 31.1) centre (31.6, 31.6) ccw
  arc A248 (45.1, 44.6) -> (44.6, 45.1) centre (44.6, 44.6) ccw
  arc A249 (31.6, 45.1) -> (31.1, 44.6) centre (31.6, 44.6) ccw
  line L262 (60.15, 32.1) -> (54.15, 32.1)
  line L263 (60.65, 32.6) -> (60.65, 45.625)
  line L264 (53.65, 32.6) -> (53.65, 45.625)
  arc A250 (60.15, 32.1) -> (60.65, 32.6) centre (60.15, 32.6) ccw
  arc A251 (53.65, 32.6) -> (54.15, 32.1) centre (54.15, 32.6) ccw
  line L265 (22.05, 32.1) -> (17.025, 32.1)
  line L266 (22.05, 47.1) -> (16.05, 47.1)
  line L267 (22.55, 32.6) -> (22.55, 46.6)
  line L268 (15.55, 45.6) -> (15.55, 46.6)
  arc A252 (22.05, 32.1) -> (22.55, 32.6) centre (22.05, 32.6) ccw
  arc A253 (22.55, 46.6) -> (22.05, 47.1) centre (22.05, 46.6) ccw
  arc A254 (16.05, 47.1) -> (15.55, 46.6) centre (16.05, 46.6) ccw
  line L269 (-12.55, 31.1) -> (-25.55, 31.1)
  line L270 (-12.55, 45.1) -> (-25.55, 45.1)
  line L271 (-12.05, 31.6) -> (-12.05, 44.6)
  line L272 (-26.05, 31.6) -> (-26.05, 44.6)
  arc A255 (-12.55, 31.1) -> (-12.05, 31.6) centre (-12.55, 31.6) ccw
  arc A256 (-26.05, 31.6) -> (-25.55, 31.1) centre (-25.55, 31.6) ccw
  arc A257 (-12.05, 44.6) -> (-12.55, 45.1) centre (-12.55, 44.6) ccw
  arc A258 (-25.55, 45.1) -> (-26.05, 44.6) centre (-25.55, 44.6) ccw
  line L273 (2.025, 32.1) -> (-3, 32.1)
  line L274 (3, 47.1) -> (-3, 47.1)
  line L275 (3.5, 45.6) -> (3.5, 46.6)
  line L276 (-3.5, 32.6) -> (-3.5, 46.6)
  arc A259 (-3.5, 32.6) -> (-3, 32.1) centre (-3, 32.6) ccw
  arc A260 (3.5, 46.6) -> (3, 47.1) centre (3, 46.6) ccw
  arc A261 (-3, 47.1) -> (-3.5, 46.6) centre (-3, 46.6) ccw
  line L277 (-35.1, 32.1) -> (-41.1, 32.1)
  line L278 (-34.6, 32.6) -> (-34.6, 45.625)
  line L279 (-41.6, 32.6) -> (-41.6, 45.625)
  arc A262 (-35.1, 32.1) -> (-34.6, 32.6) centre (-35.1, 32.6) ccw
  arc A263 (-41.6, 32.6) -> (-41.1, 32.1) centre (-41.1, 32.6) ccw
  line L280 (-55.4125, 31.1) -> (-68.4125, 31.1)
  line L281 (-55.4125, 45.1) -> (-68.4125, 45.1)
  line L282 (-54.9125, 31.6) -> (-54.9125, 44.6)
  line L283 (-68.9125, 31.6) -> (-68.9125, 44.6)
  arc A264 (-55.4125, 31.1) -> (-54.9125, 31.6) centre (-55.4125, 31.6) ccw
  arc A265 (-68.9125, 31.6) -> (-68.4125, 31.1) centre (-68.4125, 31.6) ccw
  arc A266 (-54.9125, 44.6) -> (-55.4125, 45.1) centre (-55.4125, 44.6) ccw
  arc A267 (-68.4125, 45.1) -> (-68.9125, 44.6) centre (-68.4125, 44.6) ccw
  line L284 (-79.225, 31.1) -> (-92.225, 31.1)
  line L285 (-79.225, 45.1) -> (-92.225, 45.1)
  line L286 (-78.725, 31.6) -> (-78.725, 44.6)
  line L287 (-92.725, 31.6) -> (-92.725, 44.6)
  arc A268 (-79.225, 31.1) -> (-78.725, 31.6) centre (-79.225, 31.6) ccw
  arc A269 (-92.725, 31.6) -> (-92.225, 31.1) centre (-92.225, 31.6) ccw
  arc A270 (-78.725, 44.6) -> (-79.225, 45.1) centre (-79.225, 44.6) ccw
  arc A271 (-92.225, 45.1) -> (-92.725, 44.6) centre (-92.225, 44.6) ccw
  line L288 (140.875, -47.625) -> (-140.875, -47.625)
  line L289 (142.875, 45.625) -> (142.875, -45.625)
  line L290 (-142.875, 45.625) -> (-142.875, -45.625)
  line L291 (137.4688, 26.05) -> (137.3817, 26.05)
  line L292 (129.3817, 26.05) -> (124.4687, 26.05)
  line L293 (116.0375, 26.05) -> (113.5057, 26.05)
  line L294 (105.5057, 26.05) -> (103.0375, 26.05)
  line L295 (-107.8, -31.1) -> (-107.887, -31.1)
  line L296 (-115.887, -31.1) -> (-120.8, -31.1)
  line L297 (-126.85, -31.1) -> (-131.763, -31.1)
  line L298 (-139.763, -31.1) -> (-139.85, -31.1)
  line L299 (21.7216, 49.625) -> (-2.6716, 49.625)
  line L300 (140.875, 47.625) -> (62.65, 47.625)
  line L301 (51.65, 47.625) -> (28.0552, 47.625)
  line L302 (-8.8534, 47.625) -> (-32.6, 47.625)
  line L303 (-43.6, 47.625) -> (-140.875, 47.625)
  arc A272 (53.65, 45.625) -> (51.65, 47.625) centre (51.65, 45.625) ccw
  arc A273 (62.65, 47.625) -> (60.65, 45.625) centre (62.65, 45.625) ccw
  arc A274 (-32.6, 47.625) -> (-34.6, 45.625) centre (-32.6, 45.625) ccw
  arc A275 (-41.6, 45.625) -> (-43.6, 47.625) centre (-43.6, 45.625) ccw
  arc A276 (-140.875, 47.625) -> (-142.875, 45.625) centre (-140.875, 45.625) ccw
  arc A277 (-142.875, -45.625) -> (-140.875, -47.625) centre (-140.875, -45.625) ccw
  arc A278 (140.875, -47.625) -> (142.875, -45.625) centre (140.875, -45.625) ccw
  arc A279 (142.875, 45.625) -> (140.875, 47.625) centre (140.875, 45.625) ccw
  arc A280 (136.8817, 26.55) -> (137.3817, 26.05) centre (137.3818, 26.55) ccw
  arc A281 (129.3817, 26.05) -> (129.8817, 26.55) centre (129.3817, 26.55) ccw
  arc A282 (113.0057, 26.55) -> (113.5057, 26.05) centre (113.5057, 26.55) ccw
  arc A283 (105.5057, 26.05) -> (106.0057, 26.55) centre (105.5057, 26.55) ccw
  arc A284 (15.05, 45.1) -> (15.55, 45.6) centre (15.05, 45.6) ccw
  arc A285 (17.025, 32.1) -> (16.525, 31.6) centre (17.025, 31.6) ccw
  arc A286 (2.525, 31.6) -> (2.025, 32.1) centre (2.025, 31.6) ccw
  arc A287 (3.5, 45.6) -> (4, 45.1) centre (4, 45.6) ccw
  arc A288 (-132.263, -30.6) -> (-131.763, -31.1) centre (-131.763, -30.6) ccw
  arc A289 (-139.763, -31.1) -> (-139.263, -30.6) centre (-139.763, -30.6) ccw
  arc A290 (-115.887, -31.1) -> (-115.387, -30.6) centre (-115.887, -30.6) ccw
  arc A291 (-108.387, -30.6) -> (-107.887, -31.1) centre (-107.887, -30.6) ccw
  line L304 (-2.6716, 49.625) -> (-3.5, 49.625)
  line L305 (21.7216, 49.625) -> (22.7017, 49.625)
  line L306 (22.7017, 49.625) -> (24.3983, 49.625)
  line L307 (-3.5, 49.625) -> (-5.1966, 49.625)
  line L308 (25.8125, 49.0392) -> (26.6409, 48.2108)
  line L309 (-6.6108, 49.0392) -> (-7.4392, 48.2108)
  arc A292 (26.6409, 48.2108) -> (28.0552, 47.625) centre (28.0552, 49.625) ccw
  arc A293 (25.8125, 49.0392) -> (24.3983, 49.625) centre (24.3983, 47.625) ccw
  arc A294 (-5.1966, 49.625) -> (-6.6108, 49.0392) centre (-5.1966, 47.625) ccw
  arc A295 (-8.8534, 47.625) -> (-7.4392, 48.2108) centre (-8.8534, 49.625) ccw
  point P0 (0, 0)
  point P1 (15.55, 45.1)
  point P2 (3.5, 45.1)
  point P3 (-2.2375, 0)
  point P4 (11.6161, -6.8536)
  point P5 (25.2267, 49.625)
  point P6 (-6.025, 49.625)
  point P7 (16.525, 31.6)
  point P8 (2.525, 31.6)
  dimension "d0" = 2.2375
  dimension "d1" = 7
  dimension "d2" = 14
  dimension "d3" = 14
  dimension "d4" = 0.3535
  dimension "d5" = 5.05
  dimension "d6" = 5.05
  dimension "d7" = 13
  dimension "d8" = 14
  dimension "d9" = 12.05
  dimension "d10" = 38.1
  dimension "d11" = 15
  dimension "d12" = 26.05
  dimension "d16" = 285.75
  dimension "d17" = 142.875
  dimension "d18" = 2.525
  dimension "d24" = 0.5
  dimension "d25" = 2.525
  dimension "d26" = 2.525
  dimension "d27" = 135
  dimension "d28" = 47.625
  dimension "d29" = 135
  dimension "d30" = 2
  constraints: 620 end point, 593 point on circle, 296 centre point, 44 tangent, 26 point on line, 24 equal radius, 9 horizontal, 3 equal length, 1 collinear, 1 midpoint, 1 vertical, 1 vertical alignment
  measures "d0" distance of point (-2.238, 0) point (0, 0)
  measures "d1" distance from line of point (0, 0) L144
  measures "d2" distance between parallel lines of L145 L144
  measures "d3" distance between parallel lines of L146 L147
  measures "d4" horizontal distance of point (11.616, -6.854) A140.centre
  measures "d5" distance between parallel lines of L143 L146
  measures "d6" distance between parallel lines of L144 L89
  measures "d7" distance of L248.start L248.end
  measures "d8" distance of L267.start L267.end
  measures "d9" distance of point (15.55, 45.1) point (3.5, 45.1)
  measures "d10" distance between parallel lines of L145 L249
  measures "d11" distance between parallel lines of L265 L266
  measures "d12" distance between parallel lines of L276 L267
  measures "d16" distance between parallel lines of L289 L290
  measures "d17" distance from line of L290 point (0, 0)
  measures "d18" distance between parallel lines of L274 L299
  measures "d24" radius of A280
  measures "d25" distance of L305.end point (25.227, 49.625)
  measures "d26" distance of L304.end point (-6.025, 49.625)
  measures "d27" angle of L306 L308
  measures "d28" distance from line of L302 point (0, 0)
  measures "d29" angle of L307 L309
  measures "d30" radius of A292
extrude "Extrusion1" add sketch "Sketch1" along normal blind 1.5
sketch "Sketch2" plane through (0, 1.5, 0) normal (0, 1, 0) x (1, 0, 0)
  line L0 (-119.5375, -48.1) -> (100.4875, -48.1)
  line L1 (143.35, 48.1) -> (-143.35, 48.1)
  line L2 (-143.35, 48.1) -> (-143.35, -29.05)
  line L3 (-139.85, 45.1) -> (-126.85, 45.1) projected
  line L4 (-98.275, -45.1) -> (-111.275, -45.1) projected
  line L5 (-140.35, 31.6) -> (-140.35, 44.6) projected
  line L6 (140.35, -12.55) -> (140.35, -25.55) projected
  line L7 (-143.35, -29.05) -> (-119.5375, -29.05)
  line L8 (-119.5375, -29.05) -> (-119.5375, -48.1)
  line L9 (-113.5057, -26.05) -> (-129.3817, -26.05) projected
  line L10 (142.875, -45.625) -> (142.875, 45.625) projected
  line L11 (142.875, -29.05) -> (100.4875, -29.05)
  line L12 (100.4875, -29.05) -> (100.4875, -48.1)
  line L13 (139.85, -26.05) -> (126.85, -26.05) projected
  line L14 (92.225, -45.1) -> (79.225, -45.1) projected
  line L15 (-146.35, 55.1) -> (-146.35, -55.1)
  line L16 (-146.35, -55.1) -> (146.35, -55.1)
  line L17 (146.35, -55.1) -> (146.35, 55.1)
  line L18 (146.35, 55.1) -> (-146.35, 55.1)
  line L19 (143.35, -29.05) -> (143.35, 48.1)
  line L20 (143.35, -29.05) -> (142.875, -29.05)
  point P0 (0, 0)
  point P1 (-104.775, -45.1)
  point P2 (85.725, -45.1)
  dimension "d33" = 3
  dimension "d34" = 3
  dimension "d35" = 3
  dimension "d37" = 3
  dimension "d38" = 14.7625
  dimension "d39" = 3
  dimension "d40" = 14.7625
  dimension "d41" = 3
  dimension "d42" = 7
  dimension "d44" = 7
  dimension "d45" = 3
  dimension "d46" = 3
  constraints: 26 end point, 8 perpendicular, 3 horizontal, 2 midpoint, 2 point on line, 2 vertical
  measures "d33" distance between parallel lines of L1 L3
  measures "d34" distance between parallel lines of L0 L4
  measures "d35" distance between parallel lines of L2 L5
  measures "d37" distance between parallel lines of L7 L9
  measures "d38" distance from line of L8 point (-104.775, -45.1)
  measures "d39" distance between parallel lines of L13 L11
  measures "d40" distance from line of point (85.725, -45.1) L12
  measures "d41" distance between parallel lines of L15 L2
  measures "d42" distance between parallel lines of L18 L1
  measures "d44" distance between parallel lines of L16 L0
  measures "d45" distance between parallel lines of L6 L19
  measures "d46" distance between parallel lines of L19 L17
extrude "Extrusion2" add sketch "Sketch2" along normal blind 7.5 separate body
sketch "Sketch3" plane through (146.35, 1.5, 55.1) normal (1, 0, 0) x (0, 0, -1)
  line L0 (0, 0) -> (0, -10.5)
  line L1 (0, 7.5) -> (110.2, 7.5) projected
  line L2 (0, 0) -> (110.2, 0) projected
  line L3 (110.2, 0) -> (110.2, -7.5)
  line L4 (0, -10.5) -> (9.9255, -11.7187)
  arc A0 (9.9255, -11.7187) -> (55.5786, -8.8926) centre (25.1591, 112.3496) ccw
  arc A1 (110.2, -7.5) -> (55.5786, -8.8926) centre (85.9981, -130.1347) ccw
  line L5 (9.475, -1.5) -> (100.725, -1.5) construction
  line L6 (20.8914, -1.5) -> (20.8914, -11.7187) construction
  point P0 (55.1, -1.5)
  dimension "d49" = 18
  dimension "d50" = 15
  dimension "d51" = 97
  dimension "d54" = 10
  dimension "d55" = 125
  dimension "d56" = 125
  constraints: 8 end point, 4 point on circle, 3 vertical, 2 centre point, 2 tangent, 1 point on line
  measures "d49" distance from line of L1 L0.end
  measures "d50" distance from line of L3.end L1
  measures "d51" angle of L4 L0
  measures "d54" distance of L0.end L4.end
  measures "d55" radius of A0
  measures "d56" radius of A1
body "Solid173"
